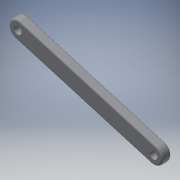
# Autodesk Inventor part: Lift Arm Upper
Saved by Autodesk Inventor 2017 (Build 210142000, 142)
## iProperties
Created: 2015-06-06
Part Number: Lift Arm Upper
Material: Generic
Document SubType Name: Modeling
Designer: Dale
Density: 1 g/cm^3
Appearance: Default
Author: Dale
## iProperties of the stored document Lift Arm Upper_3DPrint.ipt
Created: 2017-08-20
Part Number: Lift Arm Upper_3DPrint
Material: Generic
Document SubType Name: Modeling
Designer: Dale
Density: 1 g/cm^3
Appearance: Default
Author: Dale
Autodesk Inventor part; units mm, degrees
ref_plane "YZ Plane" through (0, 0, 0) normal (1, 0, 0) x (0, 1, 0)
ref_plane "XZ Plane" through (0, 0, 0) normal (0, 1, 0) x (-1, 0, 0)
ref_plane "XY Plane" through (0, 0, 0) normal (0, 0, 1) x (1, 0, 0)
sketch "Sketch6" plane through (0, 0, 0) normal (0, 0, 1) x (1, 0, 0)
  line L0 (0, 0) -> (5.6775, 19.1772)
  line L1 (5.6775, 19.1772) -> (176.8547, -31.5002)
  line L2 (176.8547, -31.5002) -> (171.1772, -50.6775)
  line L3 (171.1772, -50.6775) -> (0, 0)
  circle A0 centre (12.4274, 6.7499) radius 4
  circle A1 centre (164.4274, -38.2501) radius 4
  dimension "d48" = 20
  dimension "d50" = 8
  dimension "d51" = 10
  dimension "d52" = 10
  dimension "d53" = 10
  dimension "d54" = 10
  dimension "d55" = 45
  dimension "d56" = 152
  constraints: 8 end point, 2 centre point, 2 parallel, 1 equal radius, 1 perpendicular
  measures "d48" distance of L0.start L0.end
  measures "d50" diameter of A0
  measures "d51" distance from line of L3 A0.centre
  measures "d52" distance from line of A0.centre L0
  measures "d53" distance from line of L2 A1.centre
  measures "d54" distance from line of L3 A1.centre
  measures "d55" vertical distance of A1.centre A0.centre
  measures "d56" horizontal distance of A1.centre A0.centre
extrude "Extrusion5" add sketch "Sketch6" along normal blind 10
fillet "Fillet5" radius 10 4 edges at (5.6775, 19.1772, 5) (0, 0, 5) (176.8547, -31.5002, 5) (171.1772, -50.6775, 5)
fillet "Fillet6" radius 2 6 edges at (173.215, -33.4771, 0) (85.5886, -25.3387, 0) (91.2661, -6.1615, 0) (85.5886, -25.3387, 10) (91.2661, -6.1615, 10) (7.6544, 15.5375, 0)
fillet "Fillet7" radius 0.5 4 edges at (160.4274, -38.2501, 0) (8.4274, 6.7499, 0) (8.4274, 6.7499, 10) (160.4274, -38.2501, 10)
body "Solid3"
